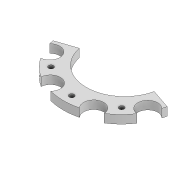
# Autodesk Inventor part: Plunger Holder
Saved by Autodesk Inventor 2020 (Build 240168000, 168)
## iProperties
Created: 2020-10-11
Part Number: Plunger Holder
Material: Generic
Document SubType Name: Modeling
Designer: ferrerx
Density: 1 g/cm^3
Appearance: Default
Author: ferrerx
Autodesk Inventor part; units mm, degrees
ref_plane "YZ Plane" through (0, 0, 0) normal (1, 0, 0) x (0, 1, 0)
ref_plane "XZ Plane" through (0, 0, 0) normal (0, 1, 0) x (-1, 0, 0)
ref_plane "XY Plane" through (0, 0, 0) normal (0, 0, 1) x (1, 0, 0)
sketch "Sketch1" plane through (0, 0, 0) normal (0, 1, 0) x (-1, 0, 0)
  line L0 (-22.5529, -44.0141) -> (22.4471, -44.0141)
  line L1 (-22.5529, -44.0141) -> (22.4471, -44.0141)
  line L2 (22.4471, 2.9859) -> (22.4471, -44.0141)
  line L3 (22.4471, 2.9859) -> (12.4471, 2.9859)
  line L4 (-22.5529, 2.9859) -> (-22.5529, -44.0141)
  line L5 (-22.5529, 2.9859) -> (-12.4471, 2.9859)
  arc A0 (-12.4471, 2.9859) -> (12.4471, 2.9859) centre (0, 4.1349) ccw
  circle A1 centre (-18.0529, -7.0141) radius 1.95
  circle A2 centre (-18.0529, -7.0141) radius 1.95
  circle A3 centre (17.9471, -7.0141) radius 1.95
  circle A4 centre (17.9471, -7.0141) radius 1.95
  circle A5 centre (0, -32.0141) radius 5.1
  circle A6 centre (-18.0529, -24.0142) radius 2
  circle A7 centre (-18, -40.0141) radius 2
  circle A8 centre (18, -40.0141) radius 2
  circle A9 centre (17.9471, -24.0142) radius 2
  line L6 (0, 4.1349) -> (0, -32.0141) construction
  point P0 (0, 0)
  dimension "d0" = 45
  dimension "d3" = 10
  dimension "d4" = 12.5
  dimension "d7" = 4.5
  dimension "d8" = 10
  dimension "d9" = 12
  dimension "d10" = 4
  dimension "d11" = 16
  dimension "d12" = 36
  dimension "d13" = 16
  dimension "d14" = 4.5
  dimension "d15" = 18
  dimension "d17" = 4.5
  dimension "d19" = 4
  dimension "d20" = 4
  dimension "d21" = 4
  dimension "d22" = 4
  dimension "d23" = 4
  dimension "d29" = 47
  dimension "d33" = 4.5
  dimension "d34" = 10
  constraints: 14 end point, 10 centre point, 3 coincident, 3 vertical, 2 collinear, 2 point on circle, 1 horizontal, 1 point on line
  measures "d0" distance of L0.start L0.end
  measures "d3" distance of L2.start L3.end
  measures "d4" radius of A0
  measures "d7" distance from line of L4 A1.centre
  measures "d8" distance from line of L5 A1.centre
  measures "d9" distance from line of L1 L6.end
  measures "d10" diameter of A7
  measures "d11" distance of A6.centre A7.centre
  measures "d12" distance of A8.centre A7.centre
  measures "d13" distance of A9.centre A8.centre
  measures "d14" distance from line of L2 A9.centre
  measures "d15" horizontal distance of A8.centre L6.end
  measures "d17" distance from line of L4 A6.centre
  measures "d19" diameter of A9
  measures "d20" diameter of A8
  measures "d21" diameter of A6
  measures "d22" distance from line of L0 A8.centre
  measures "d23" distance from line of L0 A7.centre
  measures "d29" distance between parallel lines of L0 L3
  measures "d33" distance from line of L2 A3.centre
  measures "d34" distance from line of L3 A3.centre
extrude "Extrusion1" add sketch "Sketch1" along normal blind 5
fillet "Fillet3" [suppressed]
fillet "Fillet4" [suppressed]
sketch "Sketch5" plane through (0, 5, 0) normal (0, 1, 0) x (1, 0, 0)
  arc A0 (12.4471, -2.9859) -> (-12.4471, -2.9859) centre (0, -4.1349) ccw projected
  arc A1 (12.4471, -2.9859) -> (-12.4471, -2.9859) centre (0, -4.1349) ccw
  line L0 (12.4471, -2.9859) -> (-12.4471, -2.9859)
  circle A2 centre (18.0529, 7.0141) radius 1.95 projected
  circle A3 centre (18.0529, 7.0141) radius 1.95
  circle A4 centre (-17.9471, 7.0141) radius 1.95 projected
  circle A5 centre (-17.9471, 7.0141) radius 1.95
  point P0 (0, 0)
  constraints: 3 centre point, 2 coincident, 2 end point, 2 point on circle, 1 concentric, 1 horizontal
extrude "Extrusion4" add sketch "Sketch5" against normal blind 5
sketch "Sketch8" plane through (0, 5, 0) normal (0, 1, 0) x (1, 0, 0)
  arc A0 (-25.3055, 28.046) -> (25.3055, 28.046) centre (0, 32) ccw
  arc A1 (-34.2883, 25.0481) -> (34.2883, 25.0481) centre (0, 32) ccw
  line L0 (-22.4471, -2.9859) -> (22.5529, -2.9859) projected
  line L1 (-22.4471, 44.0141) -> (-22.4471, -2.9859) projected
  line L2 (-22.4471, 29) -> (-34.2883, 25.0481)
  circle A2 centre (0, 32.0141) radius 5.1 projected
  line L3 (0, 32.0141) -> (0, 0) construction
  line L4 (-22.4471, 29) -> (-22.4471, 19.666)
  line L5 (34.2883, 25.0481) -> (22.5529, 29)
  line L6 (22.5529, -2.9859) -> (22.5529, 44.0141) projected
  line L7 (22.5529, 29) -> (22.5529, 19.8606)
  constraints: 10 end point, 6 point on circle, 5 point on line, 2 centre point, 1 coincident, 1 symmetric about line, 1 tangent, 1 vertical
extrude "Extrusion5" add sketch "Sketch8" against normal blind 5 contours L2 L1 A0 | A0 L1 A1 L2 | A0 L6 A1 L1 | L6 L5 A1
sketch "Sketch9" plane through (0, 5, 0) normal (0, 1, 0) x (1, 0, 0)
  circle A0 centre (0, 32) radius 34.9859
  line L0 (-22.4471, -2.9859) -> (22.5529, -2.9859) projected
  line L1 (22.5529, -2.9859) -> (22.5529, 5.2534) projected
  line L2 (22.5529, 5.2534) -> (22.5529, -2.9859)
  line L3 (22.5529, -2.9859) -> (-22.4471, -2.9859)
  line L4 (-22.4471, -2.9859) -> (-22.4471, 5.1645)
  point P0 (0, 0)
  point P1 (0, -2.9859)
  constraints: 6 end point, 2 collinear, 1 centre point, 1 point on circle, 1 tangent, 1 vertical
sketch "Sketch6" plane through (0, 5, 0) normal (0, 1, 0) x (1, 0, 0)
  circle A0 centre (0, 32.0141) radius 5.1 projected
  circle A1 centre (0, 32.0141) radius 32.5 construction
  line L0 (0, 32.0141) -> (0, -0.4859) construction
  line L1 (0, 32.0141) -> (-13.7351, 2.5591) construction
  line L2 (0, 32.0141) -> (-29.455, 18.279) construction
  circle A2 centre (-13, 2.2273) radius 6
  circle A3 centre (-29.455, 18.279) radius 6
  circle A4 centre (13, 2.2273) radius 6
  circle A5 centre (29.455, 18.279) radius 6
  point P0 (0, 0)
  dimension "d49" = 65
  dimension "d50" = 12
  dimension "d51" = 12
  dimension "d52" = 25
  dimension "d53" = 40
  constraints: 6 end point, 5 centre point, 4 point on circle, 2 coincident, 2 symmetric about line, 1 vertical, 2 other
  measures "d49" diameter of A1
  measures "d50" diameter of A3
  measures "d51" diameter of A2
  measures "d52" angle of L1 L0
  measures "d53" angle of L1 L2
extrude "Extrusion6" cut sketch "Sketch9" against normal blind 5 contours A0 L0 L4 | L1 L0 A0
extrude "Extrusion7" cut sketch "Sketch6" against normal blind 5 contours A2 | A3 | A4 | A5
sketch "Sketch10" plane through (0, 5, 0) normal (0, 1, 0) x (1, 0, 0)
  arc A0 (18.9875, 2.6148) -> (8.6459, -1.9008) centre (13, 2.2273) ccw projected
  circle A1 centre (13, 2.2273) radius 8.25 construction
  arc A2 (-8.6459, -1.9008) -> (-18.9875, 2.6148) centre (-13, 2.2273) ccw projected
  circle A3 centre (-13, 2.2273) radius 8.25 construction
  arc A4 (-28.9147, 12.3034) -> (-33.6819, 22.5373) centre (-29.455, 18.279) ccw projected
  circle A5 centre (-29.455, 18.279) radius 8.25 construction
  arc A6 (33.6819, 22.5373) -> (28.9147, 12.3034) centre (29.455, 18.279) ccw projected
  circle A7 centre (29.455, 18.279) radius 8.25 construction
  circle A8 centre (0, 32.0141) radius 5.1 projected
  circle A9 centre (0, 32.0141) radius 30 construction
  circle A10 centre (21.2132, 10.8009) radius 1.5
  circle A11 centre (0, 2.0141) radius 1.5
  circle A12 centre (-21.2132, 10.8009) radius 1.5
  line L0 (21.2132, 10.8009) -> (0, 32.0141) construction
  line L1 (0, 32.0141) -> (0, 2.0141) construction
  line L2 (0, 32.0141) -> (-21.2132, 10.8009) construction
  point P0 (0, 0)
  dimension "d60" = 16.5
  dimension "d61" = 16.5
  dimension "d62" = 16.5
  dimension "d63" = 16.5
  dimension "d64" = 60
  dimension "d65" = 3
  dimension "d66" = 3
  dimension "d67" = 3
  dimension "d68" = 45
  constraints: 8 centre point, 6 end point, 5 coincident, 3 point on circle, 1 perpendicular, 1 vertical
  measures "d60" diameter of A7
  measures "d61" diameter of A1
  measures "d62" diameter of A3
  measures "d63" diameter of A5
  measures "d64" diameter of A9
  measures "d65" diameter of A10
  measures "d66" diameter of A11
  measures "d67" diameter of A12
  measures "d68" angle of L1 L0
extrude "Extrusion8" cut sketch "Sketch10" against normal blind 10 contours A10 | A11 | A12
sketch "Sketch11" plane through (0, 5, 0) normal (0, 1, 0) x (1, 0, 0)
  line L0 (22.5529, 29) -> (22.5529, 44.0141) projected
  arc A0 (-22.4471, 29) -> (22.5529, 29) centre (0.0529, 33.7697) ccw
  line L1 (22.5529, 29) -> (22.5529, 44.0141)
  line L2 (22.5529, 44.0141) -> (-22.4471, 44.0141) projected
  line L3 (-22.4471, 44.0141) -> (-22.4471, 29)
  point P0 (0, 0)
  dimension "d71" = 23
  constraints: 4 end point, 2 point on circle, 1 centre point, 1 perpendicular, 1 vertical
  measures "d71" radius of A0
extrude "Extrusion9" cut sketch "Sketch11" against normal blind 10
body "Solid1"
